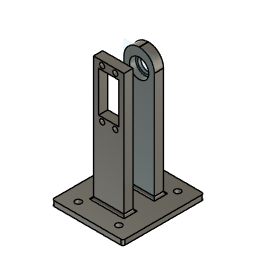
Pos15-16-35 Conjunto Lateral (Autodesk Fusion 360 design; units mm, degrees)
Autodesk Fusion 360 part; units mm, degrees
sketch "Boceto1" plane through (0, 0, 0) normal (0, 0, 1) x (1, 0, 0)
  line L0 (-35, 40) -> (35, 40)
  line L1 (35, 40) -> (35, -40)
  line L2 (35, -40) -> (-35, -40)
  line L3 (-35, -40) -> (-35, 40)
  dimension "d1" = 70
  dimension "d2" = 80
  dimension "d3" = 40
  dimension "d4" = 35
  constraint horizontal L0
  constraint vertical L1
  constraint horizontal L2
  constraint vertical L3
  measures "d1" distance of L0.start L0.end
  measures "d2" distance of L0.start L2.end
  measures "d3" distance of origin L0
  measures "d4" distance of origin L3
extrude "Extruir1" add sketch "Boceto1" along normal blind 5
fillet "Empalme1" radius 2 4 edges at (-35, -40, 2.5) (-35, 40, 2.5) (35, 40, 2.5) (35, -40, 2.5)
sketch "Boceto2" plane through (0, 0, 5) normal (0, 0, 1) x (-1, 0, 0)
  arc A0 (-33, 40) -> (-35, 38) centre (-33, 38) ccw
  line L0 (-35, 38) -> (-35, -38)
  arc A1 (-35, -38) -> (-33, -40) centre (-33, -38) ccw
  line L1 (-33, -40) -> (33, -40)
  arc A2 (33, -40) -> (35, -38) centre (33, -38) ccw
  line L2 (35, -38) -> (35, 38)
  arc A3 (35, 38) -> (33, 40) centre (33, 38) ccw
  line L3 (33, 40) -> (-33, 40)
  circle A4 centre (20, 29) radius 3
  dimension "d9" = 6
  dimension "d10" = 20
  dimension "d11" = 29
  measures "d9" diameter of A4
  measures "d10" horizontal distance of origin A4.centre
  measures "d11" vertical distance of origin A4.centre
extrude "Extruir2" cut sketch "Boceto2" against normal blind 15 contours A4
pattern_linear "Patrón R1" count 2 spacing 40 along (1, 0, 0) count 2 spacing 58 along (0, 1, 0) of "Extruir2"
sketch "Boceto3" plane through (0, 0, 5) normal (0, 0, 1) x (-1, 0, 0)
  circle A0 centre (-20, -29) radius 3
  circle A1 centre (20, -29) radius 3
  circle A2 centre (-20, 29) radius 3
  circle A3 centre (20, 29) radius 3
  arc A4 (-33, 40) -> (-35, 38) centre (-33, 38) ccw
  line L0 (-35, 38) -> (-35, -38)
  arc A5 (-35, -38) -> (-33, -40) centre (-33, -38) ccw
  line L1 (-33, -40) -> (33, -40)
  arc A6 (33, -40) -> (35, -38) centre (33, -38) ccw
  line L2 (35, -38) -> (35, 38)
  arc A7 (35, 38) -> (33, 40) centre (33, 38) ccw
  line L3 (33, 40) -> (-33, 40)
  line L4 (15, -20) -> (-15, -20)
  line L5 (-15, -20) -> (-15, -11)
  line L6 (-15, -11) -> (15, -11)
  line L7 (15, -11) -> (15, -20)
  point P0 (0, -11)
  point P1 (0, -20)
  point P2 (15, -15.5)
  dimension "d18" = 30
  dimension "d20" = 9
  dimension "d21" = 11
  constraint horizontal L4
  constraint vertical L5
  constraint horizontal L6
  constraint vertical L7
  constraint midpoint L6 P0
  constraint midpoint L4 P1
  constraint midpoint L7 P2
  constraint vertical origin P0
  measures "d18" distance of L4.start L4.end
  measures "d20" distance of L4.end L5.end
  measures "d21" distance of origin L6
extrude "Extruir3" add sketch "Boceto3" along normal blind 122 contours L4 L5 L6 L7
sketch "Boceto4" plane through (0, 11, 0) normal (0, -1, 0) x (1, 0, 0)
  line L0 (-15, 5) -> (15, 5)
  line L1 (15, 5) -> (15, 127)
  line L2 (15, 127) -> (-15, 127)
  line L3 (-15, 127) -> (-15, 5)
pattern_linear "Patrón R2" count 2 spacing 30 along (0, -1, 0) of "Extruir3"
fillet "Empalme2" chord length 21 2 edges at (15, 15.5, 127) (-15, 15.5, 127)
sketch "Boceto5" plane through (0, 11, 105) normal (0, -1, 0) x (1, 0, 0)
  circle A0 centre (0, 4) radius 9.5
  point P0 (15, -100)
  dimension "d26" = 19
  dimension "d34" = 104
  constraint vertical origin A0.centre
  measures "d26" diameter of A0
  measures "d34" vertical distance of A0.centre P0
extrude "Extruir4" cut sketch "Boceto5" against normal blind 6
sketch "Boceto6" plane through (0, 11, 0) normal (0, -1, 0) x (1, 0, 0)
  circle A0 centre (0, 109) radius 7.5
  point P0 (15, 5)
  dimension "d35" = 104
  dimension "d36" = 15
  constraint vertical A0.centre origin
  measures "d35" vertical distance of A0.centre P0
  measures "d36" diameter of A0
extrude "Extruir5" cut sketch "Boceto6" against normal blind 30
sketch "Boceto7" plane through (0, -19, 0) normal (0, -1, 0) x (1, 0, 0)
  line L0 (-15, 5) -> (15, 5)
  line L1 (15, 5) -> (15, 127)
  line L2 (15, 127) -> (-15, 127)
  line L3 (-15, 127) -> (-15, 5)
  line L4 (-10, 119) -> (10, 119)
  line L5 (10, 119) -> (10, 79)
  line L6 (10, 79) -> (-10, 79)
  line L7 (-10, 79) -> (-10, 119)
  circle A0 centre (-6.5, 123) radius 2.5
  circle A1 centre (6.5, 123) radius 2.5
  circle A2 centre (-6.5, 75) radius 2.5
  circle A3 centre (6.5, 75) radius 2.5
  point P0 (0, 119)
  point P1 (10, 99)
  dimension "d39" = 20
  dimension "d40" = 40
  dimension "d41" = 8
  dimension "d42" = 4
  dimension "d43" = 5
  dimension "d44" = 6.5
  dimension "d47" = 13
  dimension "d48" = -48
  constraint horizontal L4
  constraint vertical L5
  constraint horizontal L6
  constraint vertical L7
  constraint midpoint L4 P0
  constraint midpoint L5 P1
  constraint vertical origin P0
  measures "d39" distance of L4.start L4.end
  measures "d40" distance of L4.start L6.end
  measures "d41" distance of L2 L4
  measures "d42" distance of L2 A0.centre
  measures "d43" diameter of A0
  measures "d44" horizontal distance of P0 A0.centre
extrude "Extruir6" cut sketch "Boceto7" against normal blind 15 contours L4 L5 L6 L7 | A0 | A1 | A2 | A3
fillet "Empalme3" radius 2 8 edges at (15, -14.5, 5) (0, -19, 5) (-15, -14.5, 5) (0, -10, 5) (0, 11, 5) (15, 15.5, 5) (0, 20, 5) (-15, 15.5, 5)
equation "d44 = ( 13 / 2 ) * 1 mm"
